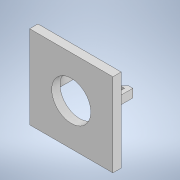
# Autodesk Inventor part: TestButtonClip
Saved by Autodesk Inventor 2020 (Build 240168000, 168)
## iProperties
Created: 2020-06-10
Part Number: TestButtonClip
Material: Generic
Document SubType Name: Modeling
Designer: Brandon
Density: 1 g/cm^3
Appearance: Default
Author: Brandon
Autodesk Inventor part; units mm, degrees
ref_plane "YZ Plane" through (0, 0, 0) normal (1, 0, 0) x (0, 1, 0)
ref_plane "XZ Plane" through (0, 0, 0) normal (0, 1, 0) x (-1, 0, 0)
ref_plane "XY Plane" through (0, 0, 0) normal (0, 0, 1) x (1, 0, 0)
sketch "Sketch1" plane through (0, 0, 0) normal (0, 0, 1) x (1, 0, 0)
  line L0 (0, 0) -> (25.4, 0)
  line L1 (25.4, 0) -> (25.4, 25.4)
  line L2 (25.4, 25.4) -> (0, 25.4)
  line L3 (0, 25.4) -> (0, 0)
  dimension "d0" = 25.4
  dimension "d1" = 25.4
  constraints: 8 end point, 2 parallel, 1 horizontal, 1 perpendicular
  measures "d0" distance of L1.end L2.end
  measures "d1" distance of L0.end L1.end
extrude "Extrusion1" add sketch "Sketch1" along normal blind 2.54
sketch "Sketch2" plane through (0, 0, 2.54) normal (0, 0, 1) x (1, 0, 0)
  circle A0 centre (12.7, 12.7) radius 5.969
  line L0 (25.4, 25.4) -> (0, 25.4) projected
  line L1 (25.4, 0) -> (25.4, 25.4) projected
  point P0 (0, 0)
  dimension "d4" = 12.7
  dimension "d5" = 12.7
  dimension "d8" = 11.938
  constraints: 1 centre point
  measures "d4" distance from line of L0 A0.centre
  measures "d5" distance from line of A0.centre L1
  measures "d8" diameter of A0
extrude "Extrusion2" cut sketch "Sketch2" against normal blind 2.54
sketch "Sketch3" plane through (0, 0, 0) normal (0, 0, -1) x (-1, 0, 0)
  line L0 (-18.796, 18.796) -> (-6.604, 18.796)
  line L1 (-6.604, 18.796) -> (-6.604, 6.604)
  line L2 (-6.604, 6.604) -> (-18.796, 6.604)
  line L3 (-18.796, 6.604) -> (-18.796, 18.796)
  line L4 (-25.4, 25.4) -> (0, 25.4) projected
  line L5 (0, 25.4) -> (0, 0) projected
  line L6 (-6.604, 13.97) -> (-5.334, 13.97)
  line L7 (-5.334, 13.97) -> (-5.334, 11.43)
  line L8 (-5.334, 11.43) -> (-6.604, 11.43)
  line L9 (-6.604, 11.43) -> (-6.604, 13.97)
  line L10 (-18.796, 13.97) -> (-20.066, 13.97)
  line L11 (-20.066, 13.97) -> (-20.066, 11.43)
  line L12 (-20.066, 11.43) -> (-18.796, 11.43)
  line L13 (-18.796, 11.43) -> (-18.796, 13.97)
  dimension "d9" = 12.192
  dimension "d10" = 12.192
  dimension "d11" = 6.604
  dimension "d12" = 6.604
  dimension "d13" = 1.27
  dimension "d14" = 1.27
  dimension "d15" = 2.54
  dimension "d16" = 11.43
  dimension "d17" = 2.54
  constraints: 24 end point, 6 parallel, 3 horizontal, 3 perpendicular, 3 point on line
  measures "d9" distance of L0.start L0.end
  measures "d10" distance of L0.end L1.end
  measures "d11" distance between parallel lines of L4 L0
  measures "d12" distance between parallel lines of L5 L1
  measures "d13" distance of L10.start L10.end
  measures "d14" distance between parallel lines of L9 L7
  measures "d15" distance between parallel lines of L8 L6
  measures "d16" distance between parallel lines of L4 L6
  measures "d17" distance between parallel lines of L10 L12
extrude "Extrusion3" add sketch "Sketch3" along normal blind 7.62 contours L3 L12 L11 L10 | L6 L7 L8 L1
sketch "Sketch4" plane through (18.796, 11.43, 0) normal (0, -1, 0) x (1, 0, 0)
  line L0 (0, -7.62) -> (1.27, -7.62) projected
  line L1 (1.27, -7.62) -> (-1.27, -7.62)
  line L2 (-1.27, -7.62) -> (-1.27, -8.89)
  line L3 (-1.27, -8.89) -> (1.27, -8.89)
  line L4 (1.27, -8.89) -> (1.27, -7.62)
  line L5 (-1.27, -7.62) -> (0, -8.89)
  line L6 (-12.192, -7.62) -> (-13.462, -7.62) projected
  line L7 (-13.462, -7.62) -> (-10.922, -7.62)
  line L8 (-10.922, -7.62) -> (-10.922, -8.89)
  line L9 (-10.922, -8.89) -> (-13.462, -8.89)
  line L10 (-13.462, -8.89) -> (-13.462, -7.62)
  line L11 (-10.922, -7.62) -> (-12.192, -8.89)
  point P0 (-18.796, 0)
  dimension "d20" = 1.27
  dimension "d21" = 2.54
  dimension "d22" = 2.54
  dimension "d23" = 1.27
  constraints: 20 end point, 4 parallel, 2 horizontal, 2 midpoint, 2 perpendicular
  measures "d20" distance of L3.end L0.end
  measures "d21" distance between parallel lines of L2 L4
  measures "d22" distance of L8.end L9.end
  measures "d23" distance between parallel lines of L6 L9
extrude "Extrusion4" add sketch "Sketch4" against normal blind 2.54 contours L0 L4 L3 L5 L1 | L7 L11 L9 L10 L6
sketch "Sketch5" plane through (18.796, 11.43, 0) normal (0, -1, 0) x (1, 0, 0)
  line L0 (6.604, 0) -> (-18.796, 0) projected
  line L1 (0.508, -5.715) -> (-12.7, -5.715)
  line L2 (-12.7, -5.715) -> (-12.7, 0)
  line L3 (-12.7, 0) -> (0.508, 0)
  line L4 (0.508, 0) -> (0.508, -5.715)
  line L5 (-13.462, 0) -> (-13.462, -8.89) projected
  dimension "d26" = 13.208
  dimension "d27" = 0.762
  dimension "d28" = 5.715
  constraints: 8 end point, 2 parallel, 1 horizontal, 1 perpendicular, 1 point on line
  measures "d26" distance of L1.start L1.end
  measures "d27" distance between parallel lines of L5 L2
  measures "d28" distance between parallel lines of L0 L1
extrude "Extrusion5" cut sketch "Sketch5" against normal blind 2.54
chamfer "Chamfer1" distance 0.508 angle 45 2 edges at (6.604, 12.7, -5.715) (18.796, 12.7, -5.715)
body "Solid1"
